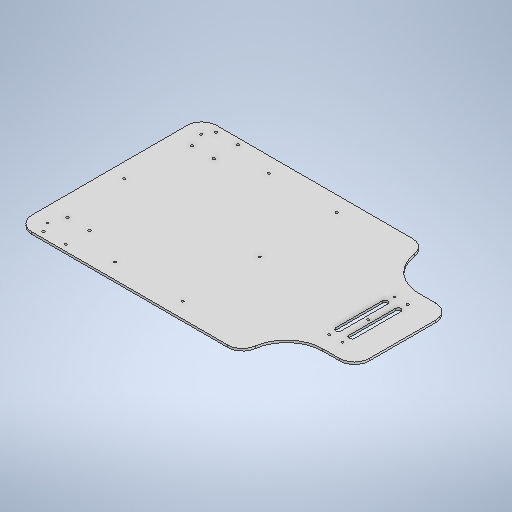
# Autodesk Inventor part: Chassis Bottom Plate
Saved by Autodesk Inventor 2025.2 (Build 292293000, 293)
## iProperties
Created: 2025-01-23
Part Number: Chassis Bottom Plate
Material: Generic
Document SubType Name: Modeling
Designer: Matt Tidd
Density: 1 g/cm^3
Appearance: Default
Author: Matt Tidd
Autodesk Inventor part; units mm, degrees
ref_plane "YZ Plane" through (0, 0, 0) normal (1, 0, 0) x (0, 1, 0)
ref_plane "XZ Plane" through (0, 0, 0) normal (0, 1, 0) x (-1, 0, 0)
ref_plane "XY Plane" through (0, 0, 0) normal (0, 0, 1) x (1, 0, 0)
sketch "Sketch1" plane through (0, 0, 0) normal (0, 1, 0) x (-1, 0, 0)
  line L0 (0, 0) -> (150, 0)
  line L1 (150, 0) -> (150, -250)
  line L2 (150, -250) -> (0, -250)
  line L3 (0, -250) -> (0, 0)
  line L4 (150, -275) -> (150, 0)
  line L5 (75, 0) -> (75, -250) construction
  line L6 (150, 0) -> (400, 0)
  line L7 (400, 0) -> (400, -250)
  line L8 (400, -250) -> (150, -250)
  line L9 (150, -250) -> (150, 0)
  line L10 (150, -250) -> (0, -250)
  line L11 (0, -250) -> (0, -200)
  line L12 (0, -200) -> (150, -200)
  line L13 (150, -200) -> (150, -250)
  line L14 (0, 0) -> (150, 0)
  line L15 (150, 0) -> (150, -50)
  line L16 (150, -50) -> (0, -50)
  line L17 (0, -50) -> (0, 0)
  line L18 (28.5, -180.5) -> (28.5, -69.5)
  line L19 (28.5, -180.5) -> (64.5, -180.5)
  line L20 (64.5, -180.5) -> (64.5, -69.5)
  line L21 (64.5, -69.5) -> (28.5, -69.5)
  line L22 (28.5, -69.5) -> (28.5, -180.5)
  line L23 (46.5, -69.5) -> (46.5, -180.5) construction
  line L24 (64.5, -125) -> (28.5, -125) construction
  circle A0 centre (46.5, -125) radius 1.5
  circle A1 centre (55.5, -80.5) radius 1.5
  circle A2 centre (55.5, -169.5) radius 1.5
  circle A3 centre (37.5, -80.5) radius 1.5
  circle A4 centre (37.5, -169.5) radius 1.5
  line L25 (55.5, -93.25) -> (55.5, -156.75) construction
  line L26 (51.75, -93.25) -> (51.75, -156.75)
  line L27 (59.25, -156.75) -> (59.25, -93.25)
  arc A5 (59.25, -93.25) -> (51.75, -93.25) centre (55.5, -93.25) ccw
  arc A6 (51.75, -156.75) -> (59.25, -156.75) centre (55.5, -156.75) ccw
  line L28 (41.25, -93.25) -> (41.25, -156.75)
  line L29 (33.75, -156.75) -> (33.75, -93.25)
  arc A7 (41.25, -93.25) -> (33.75, -93.25) centre (37.5, -93.25) ccw
  arc A8 (33.75, -156.75) -> (41.25, -156.75) centre (37.5, -156.75) ccw
  line L30 (150, -250) -> (93, -250)
  line L31 (93, -250) -> (93, 0)
  line L32 (93, 0) -> (150, 0)
  line L33 (150, 0) -> (150, -250)
  line L34 (0, -200) -> (93, -200)
  line L35 (93, -200) -> (93, -190.5)
  line L36 (93, -190.5) -> (0, -190.5)
  line L37 (0, -190.5) -> (0, -200)
  line L38 (0, -50) -> (93, -50)
  line L39 (93, -50) -> (93, -59.5)
  line L40 (93, -59.5) -> (0, -59.5)
  line L41 (0, -59.5) -> (0, -50)
  line L42 (377.5, -250) -> (377.5, 0) construction
  line L43 (377.5, -250) -> (337.5, -250) construction
  line L44 (337.5, -250) -> (337.5, -202.5) construction
  line L45 (337.5, -202.5) -> (377.5, -202.5) construction
  line L46 (377.5, -202.5) -> (377.5, -250) construction
  line L47 (377.5, 0) -> (337.5, 0) construction
  line L48 (337.5, 0) -> (337.5, -47.5) construction
  line L49 (337.5, -47.5) -> (377.5, -47.5) construction
  line L50 (377.5, -47.5) -> (377.5, 0) construction
  circle A9 centre (372.5, -242.5) radius 1.75
  circle A10 centre (342.5, -242.5) radius 1.75
  line L51 (377.5, -225) -> (337.5, -225) construction
  line L52 (377.5, -225) -> (417.5, -225) construction
  line L53 (400, -125) -> (150, -125) construction
  circle A11 centre (342.5, -210) radius 1.75
  circle A12 centre (372.5, -210) radius 1.75
  circle A13 centre (372.5, -7.5) radius 1.75
  circle A14 centre (342.5, -7.5) radius 1.75
  circle A15 centre (342.5, -40) radius 1.75
  circle A16 centre (372.5, -40) radius 1.75
  line L54 (400, 0) -> (93, 0)
  line L55 (93, 0) -> (93, 1)
  line L56 (93, 1) -> (400, 1)
  line L57 (400, 1) -> (400, 0)
  line L58 (400, -250) -> (93, -250)
  line L59 (93, -250) -> (93, -251)
  line L60 (93, -251) -> (400, -251)
  line L61 (400, -251) -> (400, -250)
  point P0 (55.5, -125)
  dimension "d0" = 150
  dimension "d1" = 250
  dimension "d9" = 250
  dimension "d10" = 50
  dimension "d11" = 50
  dimension "d14" = 36
  dimension "d15" = 3
  dimension "d16" = 3
  dimension "d18" = 7.5
  dimension "d19" = 57
  dimension "d20" = 9.5
  dimension "d21" = 9.5
  dimension "d22" = 40
  dimension "d23" = 47.5
  dimension "d24" = 40
  dimension "d25" = 47.5
  dimension "d26" = 3.5
  dimension "d27" = 3.5
  dimension "d28" = 180
  dimension "d29" = 3.5
  dimension "d30" = 3.5
  dimension "d166" = 307
  dimension "d167" = 1
  dimension "d168" = 307
  dimension "d169" = 1
  constraints: 126 end point, 25 parallel, 17 centre point, 13 horizontal, 13 perpendicular, 13 symmetric about line, 10 midpoint, 9 point on line, 8 point on circle, 4 tangent, 2 vertical, 1 collinear, 9 other
  measures "d0" distance of L1.end L2.end
  measures "d1" distance of L0.end L1.end
  measures "d9" distance of L7.end L8.end
  measures "d10" distance of L10.end L11.end
  measures "d11" distance of L14.end L15.end
  measures "d14" distance of L21.end L20.end
  measures "d15" diameter of A0
  measures "d16" diameter of A1
  measures "d18" diameter of A6
  measures "d19" distance of L31.end L32.end
  measures "d20" distance of L35.end L34.end
  measures "d21" distance of L38.end L39.end
  measures "d22" distance of L44.end L45.end
  measures "d23" distance of L43.end L44.end
  measures "d24" distance of L49.end L48.end
  measures "d25" distance of L48.end L47.end
  measures "d26" diameter of A9
  measures "d27" diameter of A10
  measures "d28" angle of L51 L52
  measures "d29" diameter of A11
  measures "d30" diameter of A12
  measures "d166" distance of L55.end L56.end
  measures "d167" distance of L54.end L55.end
  measures "d168" distance of L60.end L59.end
  measures "d169" distance of L59.end L58.end
extrude "Extrusion1" add sketch "Sketch1" along normal blind 3 contours L55 L56 L57 L6 L0 | L0 L1 L16 L31 | L6 L7 L8 L1 | L16 L1 L12 L31 | L40 L31 L36 L3 | L1 L2 L31 L12 | L61 L60 L4 L8 | L4 L60 L59 L2 | L18 L21 L20 L19
sketch "Sketch9" plane through (0, 3, 0) normal (0, 1, 0) x (1, 0, 0)
  arc A0 (-380, 250) -> (-400, 230) centre (-380, 230) ccw projected
  arc A1 (-400, 20) -> (-380, 0) centre (-380, 20) ccw projected
  line L0 (-380, 230) -> (-195, 230) construction
  line L1 (-195, 230) -> (-195, 20) construction
  line L2 (-195, 20) -> (-380, 20) construction
  line L3 (-380, 20) -> (-380, 230) construction
  circle A2 centre (-195, 230) radius 1.5
  circle A3 centre (-195, 20) radius 1.5
  circle A4 centre (-380, 20) radius 1.5
  circle A5 centre (-380, 230) radius 1.5
  line L4 (-287.5, 230) -> (-287.5, 20) construction
  line L5 (-380, 125) -> (-195, 125) construction
  circle A6 centre (-287.5, 230) radius 1.5
  circle A7 centre (-195, 125) radius 1.5
  circle A8 centre (-380, 125) radius 1.5
  circle A9 centre (-287.5, 20) radius 1.5
  point P0 (0, 0)
  dimension "d154" = 185
  dimension "d155" = 210
  dimension "d156" = 3
  dimension "d157" = 3
  dimension "d158" = 3
  dimension "d159" = 3
  dimension "d160" = 3
  dimension "d161" = 3
  dimension "d162" = 3
  dimension "d163" = 3
  constraints: 12 end point, 10 coincident, 8 centre point, 4 midpoint, 2 parallel, 1 horizontal, 1 perpendicular
  measures "d154" distance of L1.end L2.end
  measures "d155" distance of L0.end L1.end
  measures "d156" diameter of A2
  measures "d157" diameter of A3
  measures "d158" diameter of A4
  measures "d159" diameter of A5
  measures "d160" diameter of A6
  measures "d161" diameter of A7
  measures "d162" diameter of A8
  measures "d163" diameter of A9
extrude "Extrusion7" cut sketch "Sketch9" against normal blind 5
fillet "Fillet6" radius 50 2 edges at (-93, 1.5, -190.5) (-93, 1.5, -59.5)
fillet "Fillet7" radius 20 6 edges at (0, 1.5, -59.5) (0, 1.5, -190.5) (-93, 1.5, -251) (-93, 1.5, 1) (-400, 1.5, 1) (-400, 1.5, -251)
body "Solid1"
